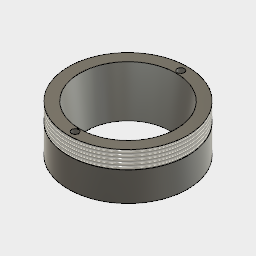
contact clamp CAM v3 (Autodesk Fusion 360 archive; units mm, degrees)
design "Collet Bottom Taper"
Autodesk Fusion 360 part; units mm, degrees
note: some values were not read from the file. Set by a fixed rule: the direction of a hole.
sketch "Sketch1" plane through (0, 0, 0) normal (0, 0, 1) x (1, 0, 0)
  line L0 (-18.15, 0) -> (-25.95, 0)
  line L1 (-25.95, 0) -> (-25.95, 12.7)
  line L2 (-25.95, 12.7) -> (-26.375, 12.7)
  line L3 (-26.375, 12.7) -> (-26.375, 20.32)
  line L4 (-26.375, 20.32) -> (-21.0058, 20.32)
  line L5 (-21.0058, 20.32) -> (-18.15, 0)
  dimension "d1" = 25.95
  dimension "d2" = 26.375
  dimension "d3" = 12.7
  dimension "d4" = 7.62
  dimension "d5" = 98
  dimension "d6" = 7.8
  dimension "d7" = 20.32
  measures "d1" distance of origin L1
  measures "d2" distance of origin L3
  measures "d3" distance of L0.end L1.end
  measures "d4" distance of L2.end L3.end
  measures "d5" angle of L0 L5
  measures "d6" distance of L0.end L0.start
  measures "d7" distance of origin L4.end
sketch "Sketch2" plane through (0, 0, 0) normal (0, 0, 1) x (1, 0, 0)
  line L0 (-18.15, 0) -> (-25.95, 0)
  line L1 (0, 0) -> (0, 22) construction
revolve "Revolve1" add sketch "Sketch1" angle 360 about axis through (0, 0, 0) along (0, 1, 0)
thread "Thread1" "ISO Metric profile 52.0 M52x1.5 6g" major diameter 51.85 minor diameter 50.1269 pitch 1.5 angle 60 resizes the face on face at (-26.3422, 15.24, -1.3147)
sketch "Sketch3" plane through (0, 20.32, 0) normal (0, 1, 0) x (-1, 0, 0)
  circle A0 centre (0, 0) radius 25.925
  circle A1 centre (0, 0) radius 21.0058
  point P0 (0, -23)
  point P1 (0, 23)
  dimension "d9" = 46
  dimension "d10" = 23
  measures "d9" distance of P0 P1
  measures "d10" distance of A0.centre P0
hole "Hole1" at (0, 20.32, -23) at (0, 20.32, 23) direction (0, -1, 0) diameter 3.1 depth 13.5 tip angle 118
equation "d1 = ( 51.9 / 2 ) * 1 mm"
equation "d2 = ( 52.75 / 2 ) * 1 mm"

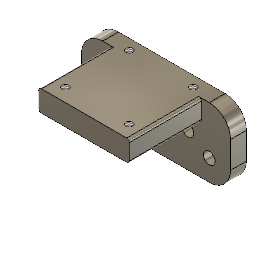
design "EX-0009723-000-XYZ-SLC-1730 z connector"
Autodesk Fusion 360 part; units mm, degrees
sketch "Sketch2" plane through (0, 0, 0) normal (0, 0, 1) x (1, 0, 0)
  arc A0 (18.5, 20) -> (18, 20.5) centre (18, 20) ccw
  line L0 (18.5, 20) -> (18.5, 8.6168)
  arc A1 (18.5, 8.6168) -> (21.6842, 3.6281) centre (24, 8.6168) ccw
  arc A2 (20, -4) -> (21.6842, 3.6281) centre (20, 0) ccw
  line L1 (20, -4) -> (0, -4)
  arc A3 (-1.6842, 3.6281) -> (0, -4) centre (0, 0) ccw
  arc A4 (-1.6842, 3.6281) -> (1.5, 8.6168) centre (-4, 8.6168) ccw
  line L2 (1.5, 8.6168) -> (1.5, 20)
  arc A5 (2, 20.5) -> (1.5, 20) centre (2, 20) ccw
  line L3 (2, 20.5) -> (18, 20.5)
  circle A6 centre (20, 0) radius 1.1
  circle A7 centre (0, 0) radius 1.1
  line L4 (24, 9) -> (-4, 9)
  line L5 (-4, 0) -> (-4, 9)
  line L6 (24, 0) -> (24, 9)
  line L7 (1.5, 9) -> (1.5, 5)
  line L8 (1.5, 5) -> (18.5, 5)
  line L9 (18.5, 5) -> (18.5, 9)
  line L10 (10, -4) -> (10, 20.5) construction
  point P0 (4, 2.5)
  point P1 (16, 2.5)
  dimension "d2" = 9
  dimension "d6" = 4
  dimension "d20" = 12
  dimension "d21" = 2.5
  constraint horizontal L4
  constraint coincident A3 L5.start
  constraint coincident A2 L6.start
  constraint tangent A2 L6
  constraint tangent A3 L5
  constraint vertical L6
  constraint vertical L5
  constraint coincident L4 L7.start
  constraint coincident L2 L7.start
  constraint perpendicular L4 L7
  constraint perpendicular L0 L8
  constraint coincident L4 L9.end
  constraint coincident L0 L9.end
  constraint perpendicular L4 L9
  constraint midpoint L1 L10.start
  constraint midpoint L3 L10.end
  constraint horizontal P0 P1
  constraint symmetric L10 P0 P1
  measures "d2" distance of A3.centre L4
  measures "d6" distance of L4 L8
  measures "d20" distance of P0 P1
  measures "d21" distance of L8 P1
ref_plane "WorkPlane1" through (0, 9, 0) normal (0, 1, 0) x (0, 0, 1)
sketch "Sketch3" plane through (0, 9, 0) normal (0, 1, 0) x (1, 0, 0)
  circle A0 centre (4, -13.5) radius 0.625
  circle A1 centre (4, -13.5) radius 0.625
  circle A2 centre (16, -13.5) radius 0.625
  circle A3 centre (16, -13.5) radius 0.625
  circle A4 centre (16, -1.5) radius 0.625
  circle A5 centre (16, -1.5) radius 0.625
  circle A6 centre (4, -1.5) radius 0.625
  circle A7 centre (4, -1.5) radius 0.625
  dimension "d4" = 12
  dimension "d5" = 12
  measures "d4" distance of A2.centre A4.centre
  measures "d5" distance of A0.centre A2.centre
extrude "Extrude1" add sketch "Sketch2" along normal blind 2.5 and the other way blind 0.5 contours L0 A1 A2 L4 L6 L9 | L0 L2 L4 L7 L8 L9 | A1 A2 L1 A3 A4 L7 L8 L9 | A3 A4 L2 L4 L5 L7
extrude "Extrude2" add sketch "Sketch2" along normal blind 16 contours L0 L2 L4 L7 L8 L9
hole "Hole1" at (4, 9, 13.5) at (16, 9, 13.5) at (16, 9, 1.5) at (4, 9, 1.5) direction (0, -1, 0) diameter 1.271 depth 6.5 tip angle 118
thread "Thread1" "ISO Metric profile 1.6 M1.6x0.35 6H"
fillet "Fillet1" radius 4 2 edges at (24, 9, 1) (-4, 9, 1)
fillet "Fillet1" radius 0.5 4 edges at (18.5, 9, 9.25) (1.5, 9, 9.25) (18.5, 5, 9.25) (1.5, 5, 9.25)
hole "Hole2" at (16, 2.5, 0) at (4, 2.5, 0) direction (0, 0, 1) diameter 2.2 depth 11 tip angle 118
hole "Hole3" at (16, 2.5, 0) at (4, 2.5, 0) direction (0, 0, -1) diameter 2.2 depth 11 tip angle 118

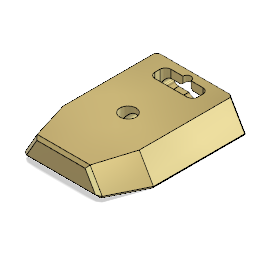
design "specimen puck"
Autodesk Fusion 360 part; units mm, degrees
sketch "Sketch1" plane through (0, 0, 0) normal (0, 0, 1) x (1, 0, 0)
  line L0 (10, 0) -> (-10, 0)
  line L1 (-10, 0) -> (-7.1132, 5)
  line L2 (-7.1132, 5) -> (7.1132, 5)
  line L3 (7.1132, 5) -> (10, 0)
  line L4 (0, 2.5) -> (0, 20)
  line L5 (-8.5566, 2.5) -> (8.5566, 2.5) construction
  line L6 (4, 3.5) -> (4, 1.5)
  line L7 (4, 3.5) -> (-4, 3.5)
  line L8 (-4, 3.5) -> (-4, 1.5)
  line L9 (-4, 1.5) -> (4, 1.5)
  dimension "d1" = 20
  dimension "d2" = 5
  dimension "d3" = 60
  dimension "d5" = 8
  dimension "d7" = 2
  measures "d1" distance of L0.start L0.end
  measures "d2" distance of L0 L2
  measures "d3" angle of L1 L3
  measures "d5" distance of L6 L8
  measures "d7" distance of L7 L9
extrude "Extrude1" add sketch "Sketch1" along normal blind 25 contours L0 L1 L2 L3 | L6 L7 L8 L9
sketch "Sketch2" plane through (0, 0, 0) normal (0, 1, 0) x (1, 0, 0)
  line L0 (-4, -4.5) -> (4, -4.5)
  line L1 (4, -4.5) -> (4, -1.5)
  line L2 (4, -1.5) -> (-4, -1.5)
  line L3 (-4, -1.5) -> (-4, -4.5)
  line L4 (10, 0) -> (-10, 0)
  line L5 (0, -1.75) -> (0, -22.5)
  point P0 (-4, 0)
  point P1 (4, 0)
  point P2 (0, -1.5)
  point P3 (0, -12.5)
  dimension "d10" = 3
  dimension "d11" = 1.5
  dimension "d27" = 12.5
  measures "d10" distance of L0 L2
  measures "d11" distance of L2 L4
  measures "d27" distance of origin P3
sketch "Sketch3" plane through (0, 5, 0) normal (0, 1, 0) x (-1, 0, 0)
  line L0 (-7.1132, 0) -> (7.1132, 0)
  line L1 (7.1132, 0) -> (7.1132, 25)
  line L2 (7.1132, 25) -> (-7.1132, 25)
  line L3 (-7.1132, 25) -> (-7.1132, 0)
  point P0 (0, 12.5)
hole "Hole1" at (0, 2.5, 0) direction (0, 0, 1) diameter 3 depth 12 tip angle 118
hole "Hole2" at (0, 0, 1.5) direction (0, 1, 0) diameter 1.5 depth 5 tip angle 118
extrude "Extrude2" cut sketch "Sketch1" along normal blind 3.5 contours L6 L7 L8 L9
extrude "Extrude3" cut sketch "Sketch2" along normal through all
ref_plane "WorkPlane1" through (0, 2.5, 17.5) normal (0, 0, 1) x (1, 0, 0)
split_face "SplitFace1" 3 faces at (8.0755, 3.3333, 8.3333) (-1.3333, 0, 18.1667) (-9.0377, 1.6667, 8.3333) by plane through (0, 2.5, 17.5) normal (0, 0, 1)
draft "Draft1" angle 15 neutral plane through (0, 2.5, 17.5) pull (0, 0, 1) 2 faces at (8.0755, 3.3333, 20) (-9.0377, 1.6667, 20)
draft "Draft2" angle 5 neutral plane through (0, 2.5, 17.5) pull (0, 0, 1) 1 faces at (-2.5598, 0, 20)
hole "Hole3" at (0, 5, 12.5) direction (0, -1, 0) diameter 3 depth 4.5 tip angle 118
chamfer "Chamfer1" distance 0.5 angle 45 10 edges at (0, 5, 25) (-6.0467, 2.8281, 25) (0, 0.6562, 25) (6.0467, 2.8281, 25) (8.6503, 0.3281, 21.25) (10, 0, 8.75) (8.5566, 2.5, 0) (-8.6503, 0.3281, 21.25) (-10, 0, 8.75) (-8.5566, 2.5, 0)
fillet "Fillet1" radius 1 10 edges at (-4, 2.5, 4.5) (-4, 4.25, 1.5) (-4, 0.75, 1.5) (4, 4.25, 1.5) (4, 0.75, 1.5) (4, 2.5, 4.5) (4, 1.5, 0.75) (4, 3.5, 0.75) (-4, 3.5, 0.75) (-4, 1.5, 0.75)

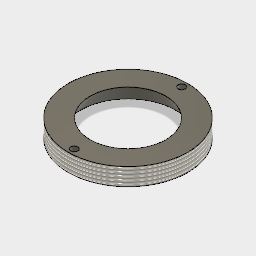
design "Collet Top Taper"
Autodesk Fusion 360 part; units mm, degrees
sketch "Sketch1" plane through (0, 0, 0) normal (0, 0, 1) x (1, 0, 0)
  line L0 (-20.7744, 0) -> (-26.35, 0)
  line L1 (-26.35, 0) -> (-26.35, 7.62)
  line L2 (-26.35, 7.62) -> (-16.375, 7.62)
  line L3 (-16.375, 7.62) -> (-20.7744, 0)
  dimension "d1" = 26.35
  dimension "d2" = 16.375
  dimension "d3" = 60
  dimension "d4" = 7.62
  dimension "d5" = 7.62
  measures "d1" distance of origin L0.end
  measures "d2" distance of origin L2.end
  measures "d3" angle of L0 L3
  measures "d4" distance of L0.end L1.end
  measures "d5" distance of origin L2.end
sketch "Sketch2" plane through (0, 0, 0) normal (0, 0, 1) x (1, 0, 0)
  line L0 (0, 0) -> (0, 1)
  line L1 (0, 1) -> (0, 14) construction
revolve "Revolve1" add sketch "Sketch1" angle 360 about axis through (0, 1, 0) along (0, 1, 0)
thread "Thread1" "ISO Metric profile 52.0 M52x1.5 6g" major diameter 51.85 minor diameter 50.1269 pitch 1.5 angle 60 resizes the face on face at (-26.2191, 2.54, -2.6236)
sketch "Sketch3" plane through (0, 7.62, 0) normal (0, 1, 0) x (-1, 0, 0)
  circle A0 centre (0, 0) radius 25.925
  circle A1 centre (0, 0) radius 16.375
  point P0 (-0.0141, -23.35)
  point P1 (-0.0141, 23.35)
  dimension "d7" = 46.7
  dimension "d8" = 23.35
  measures "d7" distance of P0 P1
  measures "d8" distance of A0.centre P0
hole "Hole1" at (0.0141, 7.62, -23.35) at (0.0141, 7.62, 23.35) direction (0, -1, 0) diameter 3.1 depth 13.5 tip angle 118
equation "d1 = ( 52.7 / 2 ) * 1 mm"
equation "d2 = ( 32.75 / 2 ) * 1 mm"
